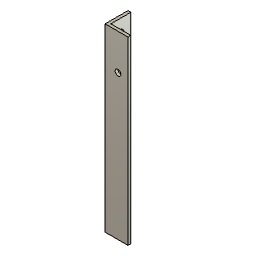
Angle 200 mm 2nd Standing Reverse v1 (Autodesk Fusion 360 design; units mm, degrees)
Autodesk Fusion 360 part; units mm, degrees
sketch "Sketch1" plane through (0, 0, 0) normal (0, 1, 0) x (1, 0, 0)
  line L0 (0, -25.4) -> (0, 0)
  line L1 (0, 0) -> (25.4, 0)
  line L2 (12.7, -12.7) -> (11.05, -11.05) construction
  line L3 (3.175, -25.4) -> (3.175, -3.175)
  line L4 (3.175, -3.175) -> (25.4, -3.175)
  line L5 (25.4, -3.175) -> (25.4, 0)
  line L6 (0, -25.4) -> (3.175, -25.4)
  dimension "d1" = 25.4
  dimension "d2" = 25.4
  dimension "d13" = 3.175
  constraint coincident L0.end L2
  constraint coincident L0.end L1.start
  constraint perpendicular L1 L5
  constraint vertical L0
  constraint horizontal L1
  measures "d1" distance of L0.end L1.end
  measures "d2" distance of L0.start L0.end
extrude "Extrude1" add sketch "Sketch1" along normal blind 200 makes body 1
hole "Hole3" at (3.175, 11.113, 14.287) direction (-1, 0, 0) diameter 6.5 end through all bodies 1
hole "Hole4" at (3.175, 185.772, 14.287) direction (-1, 0, 0) diameter 6.5 depth 30 tip angle 118 bodies 1
hole "Hole5" at (14.287, 160.312, 3.175) direction (0, 0, -1) diameter 6.5 depth 30 tip angle 118 bodies 1
mirror "Mirror2" about plane through (0, 0, 0) normal (0, 0, -1) of bodies 1 makes body 2
delete_body "RemoveBody1" bodies 1
